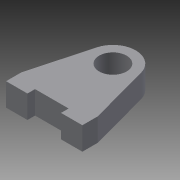
# Autodesk Inventor part: 零件4
Saved by Autodesk Inventor 2014 (Build 180170000, 170)
## iProperties
Created: 2018-10-26
Part Number: 零件4
Material: 常规
Document SubType Name: Modeling
Designer: Administrator
Density: 1 g/cm^3
Appearance: 默认
Author: Administrator
Autodesk Inventor part; units mm, degrees
ref_plane "YZ Plane" through (0, 0, 0) normal (1, 0, 0) x (0, 1, 0)
ref_plane "XZ Plane" through (0, 0, 0) normal (0, 1, 0) x (-1, 0, 0)
ref_plane "XY Plane" through (0, 0, 0) normal (0, 0, 1) x (1, 0, 0)
sketch "草图1" plane through (0, 0, 0) normal (0, 0, 1) x (1, 0, 0)
  line L0 (0, 7.9673) -> (0, -10.1658)
  circle A0 centre (0, 0) radius 9
  line L1 (-14.4802, 3.9145) -> (-25, -35)
  line L2 (14.4802, 3.9145) -> (25, -35)
  line L3 (-25, -35) -> (-25, -45)
  line L4 (-25, -45) -> (-11, -45)
  line L5 (-11, -45) -> (-11, -40)
  line L6 (-11, -40) -> (11, -40)
  line L7 (11, -40) -> (11, -45)
  line L8 (25, -45) -> (11, -45)
  line L9 (25, -35) -> (25, -45)
  arc A1 (14.4802, 3.9145) -> (-14.4802, 3.9145) centre (0, 0) ccw
  dimension "d1" = 18
  dimension "d2" = 22
  dimension "d3" = 50
  dimension "d4" = 5
  dimension "d5" = 10
  dimension "d6" = 45
  dimension "d7" = 15
  constraints: 20 end point, 6 perpendicular, 2 centre point, 2 point on circle, 2 tangent, 1 coincident, 1 concentric, 1 parallel, 1 vertical, 4 other
  measures "d1" diameter of A0
  measures "d2" distance of L5.end L6.end
  measures "d3" distance between parallel lines of L9 L3
  measures "d4" distance of L4.end L5.end
  measures "d5" distance of L1.end L3.end
  measures "d6" distance from line of point (0, 0) L4
  measures "d7" radius of A1
extrude "拉伸1" add sketch "草图1" along normal blind 15
